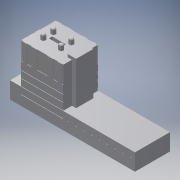
# Autodesk Inventor part: Vertigo
Saved by Autodesk Inventor 2018.3 (Build 223284000, 284)
## iProperties
Created: 2020-12-08
Part Number: Vertigo
Material: Acetal Resin, White
Document SubType Name: Modeling
Designer: daanv
Density: 1.425 g/cm^3
Appearance: Smooth - White
Author: daanv
Autodesk Inventor part; units mm, degrees
note: some values were not read from the file. Chosen so that the rebuilt part matches the saved one: pattern direction of "Rectangular Pattern3".
ref_plane "YZ Plane" through (0, 0, 0) normal (1, 0, 0) x (0, 1, 0)
ref_plane "XZ Plane" through (0, 0, 0) normal (0, 1, 0) x (-1, 0, 0)
ref_plane "XY Plane" through (0, 0, 0) normal (0, 0, 1) x (1, 0, 0)
sketch "Sketch1" plane through (0, 0, 0) normal (0, 0, 1) x (1, 0, 0)
  line L0 (0, 0) -> (100, 0)
  line L1 (100, 0) -> (100, 28.01)
  line L2 (100, 28.01) -> (0, 28.01)
  line L3 (0, 28.01) -> (0, 0)
  dimension "d0" = 100
  dimension "d1" = 28.01
  constraints: 8 end point, 2 parallel, 1 horizontal, 1 perpendicular
  measures "d0" distance of L2.end L1.end
  measures "d1" distance of L1.end L0.end
extrude "Extrusion1" add sketch "Sketch1" along normal blind 13.41
sketch "Sketch2" plane through (0, 0, 13.41) normal (0, 0, 1) x (1, 0, 0)
  line L0 (0, 0) -> (100, 0) projected
  line L1 (100, 0) -> (100, 28.01) projected
  line L2 (100, 28.01) -> (0, 28.01) projected
  line L3 (0, 28.01) -> (0, 0) projected
  line L4 (8.81, 27.7) -> (42.45, 27.7)
  line L5 (42.45, 27.7) -> (42.45, 0.31)
  line L6 (42.45, 0.31) -> (8.81, 0.31)
  line L7 (8.81, 0.31) -> (8.81, 27.7)
  dimension "d4" = 0.31
  dimension "d5" = 0.31
  dimension "d6" = 8.81
  dimension "d7" = 57.55
  dimension "d8" = 33.64
  dimension "d9" = 27.39
  constraints: 8 end point, 2 parallel, 1 horizontal, 1 perpendicular
  measures "d4" distance between parallel lines of L0 L6
  measures "d5" distance between parallel lines of L2 L4
  measures "d6" distance between parallel lines of L7 L3
  measures "d7" distance between parallel lines of L1 L5
  measures "d8" distance of L4.start L4.end
  measures "d9" distance of L4.end L5.end
extrude "Extrusion2" add sketch "Sketch2" along normal blind 31.92 contours L4 L5 L6 L7
sketch "Sketch3" plane through (0, 0, 13.41) normal (0, 0, 1) x (1, 0, 0)
  line L0 (42.45, 27.7) -> (42.45, 0.31) projected
  line L1 (42.45, 0.31) -> (8.81, 0.31) projected
  line L2 (8.81, 27.7) -> (42.45, 27.7) projected
  line L3 (42.45, 20.9) -> (45.8, 20.9)
  line L4 (45.8, 20.9) -> (45.8, 7.11)
  line L5 (45.8, 7.11) -> (42.45, 7.11)
  line L6 (42.45, 7.11) -> (42.45, 20.9)
  dimension "d12" = 6.8
  dimension "d13" = 6.8
  dimension "d14" = 3.35
  constraints: 8 end point, 2 parallel, 1 horizontal, 1 perpendicular, 1 point on line
  measures "d12" distance between parallel lines of L1 L5
  measures "d13" distance between parallel lines of L3 L2
  measures "d14" distance between parallel lines of L4 L0
extrude "Extrusion3" add sketch "Sketch3" along normal blind 34.21
sketch "Sketch4" plane through (42.45, 7.11, 45.33) normal (-1, 0, 0) x (0, 0, 1)
  line L0 (0, 0) -> (0, 13.79) projected
  line L1 (0, 0) -> (2.29, 0) projected
  line L2 (2.29, 13.79) -> (2.29, 0) projected
  line L3 (0, 13.79) -> (2.29, 13.79) projected
  point P0 (-45.33, -7.11)
extrude "Extrusion4" add sketch "Sketch4" along normal blind 3.44
sketch "Sketch5" plane through (0, 0, 0) normal (0, -1, 0) x (1, 0, 0)
  line L0 (100, 0) -> (100, 13.41) projected
  line L1 (0, 13.41) -> (100, 13.41) projected
  line L2 (97.05, 10.28) -> (95.8, 10.28)
  line L3 (95.8, 10.28) -> (95.8, 7.78)
  line L4 (95.8, 7.78) -> (97.05, 7.78)
  line L5 (97.05, 7.78) -> (97.05, 10.28)
  dimension "d19" = 2.5
  dimension "d20" = 1.25
  dimension "d21" = 1.25
  dimension "d22" = 3.13
  dimension "d23" = 2.95
  constraints: 8 end point, 2 parallel, 1 horizontal, 1 perpendicular
  measures "d19" distance of L2.end L3.end
  measures "d20" distance of L3.end L4.end
  measures "d21" distance of L2.start L2.end
  measures "d22" distance between parallel lines of L1 L2
  measures "d23" distance between parallel lines of L0 L5
extrude "Extrusion5" cut sketch "Sketch5" against normal blind 0.31
pattern_linear "Rectangular Pattern1" count 9 spacing 6.25 along (-1, 0, 0) of "Extrusion5"
sketch "Sketch6" plane through (0, 0, 0) normal (0, -1, 0) x (1, 0, 0)
  line L0 (45.8, 7.78) -> (45.8, 10.28) projected
  line L1 (0, 0) -> (100, 0) projected
  line L2 (0, 13.41) -> (100, 13.41) projected
  line L3 (42.45, 10.28) -> (8.49, 10.28)
  line L4 (8.49, 10.28) -> (8.49, 7.78)
  line L5 (8.49, 7.78) -> (42.45, 7.78)
  line L6 (42.45, 7.78) -> (42.45, 10.28)
  dimension "d29" = 3.35
  dimension "d30" = 33.96
  dimension "d31" = 3.13
  dimension "d32" = 7.78
  constraints: 8 end point, 2 parallel, 1 horizontal, 1 perpendicular
  measures "d29" distance between parallel lines of L0 L6
  measures "d30" distance of L4.end L5.end
  measures "d31" distance between parallel lines of L2 L3
  measures "d32" distance between parallel lines of L1 L5
extrude "Extrusion6" cut sketch "Sketch6" against normal blind 0.31
sketch "Sketch7" plane through (0, 28.01, 0) normal (0, 1, 0) x (1, 0, 0)
  line L0 (95.8, -7.78) -> (95.8, -10.28) projected
  line L1 (97.05, -10.28) -> (97.05, -7.78) projected
  line L2 (95.8, -10.28) -> (97.05, -10.28)
  line L3 (97.05, -10.28) -> (97.05, -7.78)
  line L4 (97.05, -7.78) -> (95.8, -7.78)
  line L5 (95.8, -7.78) -> (95.8, -10.28)
  constraints: 8 end point, 2 parallel, 1 horizontal, 1 perpendicular
extrude "Extrusion7" cut sketch "Sketch7" against normal blind 0.31
pattern_linear "Rectangular Pattern2" count 9 spacing 6.25 along (-1, 0, 0) of "Extrusion7"
sketch "Sketch8" plane through (0, 28.01, 0) normal (0, 1, 0) x (1, 0, 0)
  line L0 (8.49, -10.28) -> (42.45, -10.28) projected
  line L1 (42.45, -7.78) -> (8.49, -7.78) projected
  line L2 (42.45, -10.28) -> (8.49, -10.28)
  line L3 (8.49, -10.28) -> (8.49, -7.78)
  line L4 (8.49, -7.78) -> (42.45, -7.78)
  line L5 (42.45, -7.78) -> (42.45, -10.28)
  constraints: 8 end point, 2 parallel, 1 horizontal, 1 perpendicular
extrude "Extrusion8" cut sketch "Sketch8" against normal blind 0.31
sketch "Sketch9" plane through (0, 0, 0) normal (-1, 0, 0) x (0, 0, 1)
  line L0 (0, 28.01) -> (0, 0) projected
  line L1 (0, 28.01) -> (13.41, 28.01) projected
  line L2 (0, 0.7696) -> (5.26, 0.7696)
  line L3 (5.26, 0.7696) -> (5.26, 27.3796)
  line L4 (5.26, 27.3796) -> (2.67, 27.3796)
  line L5 (2.67, 27.3796) -> (2.67, 25.2896)
  line L6 (2.67, 25.2896) -> (0, 0.7696)
  dimension "d42" = 5.26
  dimension "d43" = 26.61
  dimension "d44" = 2.59
  dimension "d45" = 2.09
  constraints: 10 end point, 2 horizontal, 2 perpendicular, 1 point on line
  measures "d42" distance of L2.start L2.end
  measures "d43" distance of L2.end L3.end
  measures "d44" distance of L3.end L4.end
  measures "d45" distance of L4.end L5.end
extrude "Extrusion9" cut sketch "Sketch9" against normal blind 1.25
sketch "Sketch10" plane through (1.25, 0, 0) normal (-1, 0, 0) x (0, 0, 1)
  line L0 (2.67, 27.3796) -> (5.26, 27.3796) projected
  line L1 (2.67, 25.2896) -> (2.67, 27.3796) projected
  line L2 (5.26, 27.3796) -> (2.67, 27.3796)
  line L3 (2.67, 27.3796) -> (2.67, 25.2896)
  line L4 (2.67, 25.2896) -> (5.26, 25.2896)
  line L5 (5.26, 25.2896) -> (5.26, 27.3796)
  point P0 (0, 0)
  constraints: 8 end point, 2 parallel, 1 horizontal, 1 perpendicular
extrude "Extrusion10" cut sketch "Sketch10" against normal blind 1.24
sketch "Sketch11" plane through (8.81, 0.31, 13.41) normal (0, -1, 0) x (1, 0, 0)
  line L0 (33.64, 0) -> (0, 0) projected
  line L1 (0, 0) -> (0, 31.92) projected
  line L2 (33.64, 31.92) -> (33.64, 0) projected
  line L3 (0, 2.5) -> (33.64, 2.5)
  line L4 (33.64, 2.5) -> (33.64, 5.63)
  line L5 (33.64, 5.63) -> (0, 5.63)
  line L6 (0, 5.63) -> (0, 2.5)
  point P0 (-8.81, -13.41)
  dimension "d50" = 3.13
  dimension "d51" = 2.5
  constraints: 8 end point, 2 parallel, 2 point on line, 1 horizontal, 1 perpendicular
  measures "d50" distance of L4.end L3.end
  measures "d51" distance between parallel lines of L0 L3
extrude "Extrusion11" add sketch "Sketch11" along normal blind 0.31 contours L3 L1 L5 L2
pattern_linear "Rectangular Pattern3" count 2 spacing 5.63 along (0, 0, 1) of "Extrusion11"
sketch "Sketch12" plane through (8.81, 0.31, 45.33) normal (0, -1, 0) x (1, 0, 0)
  line L0 (0, -20.66) -> (33.64, -20.66) projected
  line L1 (33.64, -20.66) -> (33.64, 0) projected
  line L2 (0, -20.66) -> (0, 0) projected
  line L3 (0, -18.16) -> (33.64, -18.16)
  line L4 (33.64, -18.16) -> (33.64, -14.09)
  line L5 (33.64, -14.09) -> (0, -14.09)
  line L6 (0, -14.09) -> (0, -18.16)
  point P0 (-8.81, -45.33)
  dimension "d57" = 4.07
  dimension "d58" = 2.5
  constraints: 8 end point, 2 parallel, 2 point on line, 1 horizontal, 1 perpendicular
  measures "d57" distance of L4.end L3.end
  measures "d58" distance between parallel lines of L0 L3
extrude "Extrusion12" add sketch "Sketch12" along normal blind 0.31 contours L2 L5 L1 L3
sketch "Sketch13" plane through (8.81, 0.31, 31.24) normal (0, 0, 1) x (1, 0, 0)
  line L0 (0, 0) -> (33.64, 0) projected
  line L1 (33.64, -0.31) -> (0, -0.31) projected
  line L2 (-8.81, -0.31) -> (91.19, -0.31) projected
  line L3 (1.52, 0) -> (4.62, 0)
  line L4 (4.62, 0) -> (4.62, -0.31)
  line L5 (4.62, -0.31) -> (1.52, -0.31)
  line L6 (1.52, -0.31) -> (1.52, 0)
  line L7 (-0.32, 0) -> (33.64, 0) projected
  line L8 (8.21, 0) -> (12.82, 0)
  line L9 (12.82, 0) -> (12.82, -0.31)
  line L10 (12.82, -0.31) -> (8.21, -0.31)
  line L11 (8.21, -0.31) -> (8.21, 0)
  line L12 (21.12, 0) -> (25.73, 0)
  line L13 (25.73, 0) -> (25.73, -0.31)
  line L14 (25.73, -0.31) -> (21.12, -0.31)
  line L15 (21.12, -0.31) -> (21.12, 0)
  line L16 (29.32, 0) -> (32.42, 0)
  line L17 (32.42, 0) -> (32.42, -0.31)
  line L18 (32.42, -0.31) -> (29.32, -0.31)
  line L19 (29.32, -0.31) -> (29.32, 0)
  dimension "d61" = 3.1
  dimension "d62" = 4.61
  dimension "d63" = 4.61
  dimension "d64" = 3.1
  constraints: 32 end point, 8 parallel, 8 point on line, 4 horizontal, 4 perpendicular
  measures "d61" distance of L4.end L5.end
  measures "d62" distance of L9.end L10.end
  measures "d63" distance of L13.end L14.end
  measures "d64" distance of L17.end L18.end
extrude "Extrusion13" add sketch "Sketch13" along normal blind 14.1 contours L0 L4 L1 L6 | L0 L9 L1 L11 | L0 L13 L1 L15 | L0 L17 L1 L19
sketch "Sketch14" plane through (8.81, 27.7, 13.41) normal (0, 1, 0) x (1, 0, 0)
  line L0 (0, 0) -> (0, -31.92) projected
  line L1 (33.64, -2.5) -> (0, -2.5) projected
  line L2 (33.64, -5.63) -> (0, -5.63) projected
  line L3 (33.64, -2.5) -> (0, -2.5)
  line L4 (0, -2.5) -> (0, -5.63)
  line L5 (0, -5.63) -> (33.64, -5.63)
  line L6 (33.64, -5.63) -> (33.64, -2.5)
  line L7 (0, -8.13) -> (33.64, -8.13) projected
  line L8 (0, -11.26) -> (33.64, -11.26) projected
  line L9 (33.64, -8.13) -> (0, -8.13)
  line L10 (0, -8.13) -> (0, -11.26)
  line L11 (0, -11.26) -> (33.64, -11.26)
  line L12 (33.64, -11.26) -> (33.64, -8.13)
  line L13 (33.64, -13.76) -> (0, -13.76) projected
  line L14 (1.52, -17.83) -> (0, -17.83) projected
  line L15 (33.64, -13.76) -> (0, -13.76)
  line L16 (0, -13.76) -> (0, -17.83)
  line L17 (0, -17.83) -> (33.64, -17.83)
  line L18 (33.64, -17.83) -> (33.64, -13.76)
  point P0 (-8.81, 13.41)
  constraints: 24 end point, 6 parallel, 3 horizontal, 3 perpendicular
extrude "Extrusion14" add sketch "Sketch14" along normal blind 0.31
sketch "Sketch15" plane through (8.81, 27.7, 45.33) normal (0, 1, 0) x (1, 0, 0)
  line L0 (32.42, 14.09) -> (32.42, -0.01) projected
  line L1 (29.32, 14.09) -> (29.32, -0.01) projected
  line L2 (32.42, -0.01) -> (29.32, -0.01)
  line L3 (29.32, -0.01) -> (29.32, 14.09)
  line L4 (29.32, 14.09) -> (32.42, 14.09)
  line L5 (32.42, 14.09) -> (32.42, -0.01)
  line L6 (25.73, 0) -> (25.73, 14.09) projected
  line L7 (21.12, 14.09) -> (21.12, -0.01) projected
  line L8 (25.73, 0) -> (21.12, 0)
  line L9 (21.12, 0) -> (21.12, 14.09)
  line L10 (21.12, 14.09) -> (25.73, 14.09)
  line L11 (25.73, 14.09) -> (25.73, 0)
  line L12 (12.82, 14.09) -> (12.82, -0.01) projected
  line L13 (8.21, 14.09) -> (8.21, -0.01) projected
  line L14 (12.82, -0.01) -> (8.21, -0.01)
  line L15 (8.21, -0.01) -> (8.21, 14.09)
  line L16 (8.21, 14.09) -> (12.82, 14.09)
  line L17 (12.82, 14.09) -> (12.82, -0.01)
  line L18 (1.52, 14.09) -> (1.52, 0) projected
  line L19 (4.62, 14.09) -> (4.62, -0.01) projected
  line L20 (1.52, 0) -> (4.62, 0)
  line L21 (4.62, 0) -> (4.62, 14.09)
  line L22 (4.62, 14.09) -> (1.52, 14.09)
  line L23 (1.52, 14.09) -> (1.52, 0)
  point P0 (-8.81, 45.33)
  constraints: 32 end point, 8 parallel, 4 horizontal, 4 perpendicular
extrude "Extrusion15" add sketch "Sketch15" along normal blind 0.31
sketch "Sketch16" plane through (8.81, 0.31, 13.41) normal (-1, 0, 0) x (0, 0, 1)
  line L0 (17.82, 27.39) -> (0, 27.39)
  line L1 (0, 27.39) -> (0, 0)
  line L2 (0, 0) -> (17.82, 0)
  line L3 (17.82, 0) -> (17.82, 27.39)
  point P0 (-13.41, -0.31)
  constraints: 8 end point, 2 parallel, 1 horizontal, 1 perpendicular
extrude "Extrusion16" add sketch "Sketch16" along normal blind 0.31
sketch "Sketch17" plane through (8.81, 0.31, 45.33) normal (-1, 0, 0) x (0, 0, 1)
  line L0 (0, 27.39) -> (0, 0) projected
  line L1 (-14.09, 27.39) -> (0, 27.39) projected
  line L2 (-14.1, 27.39) -> (-14.1, 0) projected
  line L3 (0, 6.8) -> (0, 20.59) projected
  line L4 (-14.1, 15) -> (0, 15)
  line L5 (0, 15) -> (0, 10.62)
  line L6 (0, 10.62) -> (-14.1, 10.62)
  line L7 (-14.1, 10.62) -> (-14.1, 15)
  line L8 (0, 9.92) -> (-14.1, 9.92)
  line L9 (-14.1, 9.92) -> (-14.1, 5.54)
  line L10 (-14.1, 5.54) -> (0, 5.54)
  line L11 (0, 5.54) -> (0, 9.92)
  line L12 (0, 0) -> (0, 6.8) projected
  line L13 (0, 4.84) -> (-14.1, 4.84)
  line L14 (-14.1, 4.84) -> (-14.1, 0.46)
  line L15 (-14.1, 0.46) -> (0, 0.46)
  line L16 (0, 0.46) -> (0, 4.84)
  point P0 (-45.33, -0.31)
  dimension "d73" = 4.38
  dimension "d74" = 4.38
  dimension "d75" = 4.38
  dimension "d76" = 12.39
  dimension "d77" = 0.7
  dimension "d78" = 0.7
  constraints: 24 end point, 6 parallel, 6 point on line, 3 horizontal, 3 perpendicular
  measures "d73" distance of L4.end L5.end
  measures "d74" distance of L9.end L8.end
  measures "d75" distance of L14.end L13.end
  measures "d76" distance between parallel lines of L1 L4
  measures "d77" distance between parallel lines of L6 L8
  measures "d78" distance between parallel lines of L10 L13
extrude "Extrusion17" add sketch "Sketch17" along normal blind 0.31 contours L0 L6 L2 L4 | L0 L10 L2 L8 | L0 L15 L2 L13
sketch "Sketch18" plane through (0, 0, 45.33) normal (0, 0, 1) x (1, 0, 0)
  line L0 (39.01, 7.11) -> (39.01, 20.9) projected
  line L1 (42.45, 20.9) -> (42.45, 27.7) projected
  line L2 (29.93, 27.7) -> (21.63, 27.7) projected
  line L3 (8.81, 27.7) -> (8.81, 15.31) projected
  line L4 (13.91, 21.01) -> (33.91, 21.01)
  line L5 (33.91, 21.01) -> (33.91, 7.01)
  line L6 (33.91, 7.01) -> (13.91, 7.01)
  line L7 (13.91, 7.01) -> (13.91, 21.01)
  line L8 (16.7794, 19.91) -> (18.5188, 18.6463)
  line L9 (18.5188, 18.6463) -> (17.8544, 16.6015)
  line L10 (17.8544, 16.6015) -> (15.7044, 16.6015)
  line L11 (15.7044, 16.6015) -> (15.04, 18.6463)
  line L12 (15.04, 18.6463) -> (16.7794, 19.91)
  line L13 (32.7788, 18.6463) -> (32.1144, 16.6015)
  line L14 (32.1144, 16.6015) -> (29.9644, 16.6015)
  line L15 (29.9644, 16.6015) -> (29.3, 18.6463)
  line L16 (29.3, 18.6463) -> (31.0394, 19.91)
  line L17 (31.0394, 19.91) -> (32.7788, 18.6463)
  line L18 (16.7794, 11.7685) -> (18.5188, 10.5048)
  line L19 (18.5188, 10.5048) -> (17.8544, 8.46)
  line L20 (17.8544, 8.46) -> (15.7044, 8.46)
  line L21 (15.7044, 8.46) -> (15.04, 10.5048)
  line L22 (15.04, 10.5048) -> (16.7794, 11.7685)
  line L23 (31.0396, 11.7685) -> (32.779, 10.5048)
  line L24 (32.779, 10.5048) -> (32.1146, 8.46)
  line L25 (32.1146, 8.46) -> (29.9646, 8.46)
  line L26 (29.9646, 8.46) -> (29.3002, 10.5048)
  line L27 (29.3002, 10.5048) -> (31.0396, 11.7685)
  line L28 (18.41, 15.31) -> (29.41, 15.31)
  line L29 (29.41, 15.31) -> (29.41, 12.71)
  line L30 (29.41, 12.71) -> (18.41, 12.71)
  line L31 (18.41, 12.71) -> (18.41, 15.31)
  point P0 (8.5, 0.77)
  point P1 (21.63, 0.31)
  point P2 (0, 0)
  point P3 (16.7794, 18.0811)
  point P4 (31.0394, 18.0811)
  point P5 (16.7794, 9.9396)
  point P6 (31.0396, 9.9396)
  dimension "d81" = 33.64
  dimension "d82" = 26.93
  dimension "d83" = 20
  dimension "d84" = 14
  dimension "d85" = 6.69
  dimension "d86" = 6.7
  dimension "d87" = 5.1
  dimension "d88" = 5.1
  dimension "d89" = 2.15
  dimension "d90" = 1.13
  dimension "d91" = 1.1
  dimension "d92" = 2.15
  dimension "d94" = 1.1
  dimension "d95" = 12.11
  dimension "d96" = 1.1312
  dimension "d97" = 2.15
  dimension "d98" = 2.15
  dimension "d99" = 1.45
  dimension "d100" = 1.45
  dimension "d101" = 1.13
  dimension "d102" = 1.131
  dimension "d103" = 4.833
  dimension "d104" = 12.1102
  dimension "d105" = 11
  dimension "d106" = 2.6
  dimension "d107" = 4.5
  dimension "d108" = 5.7
  constraints: 56 end point, 6 horizontal, 4 parallel, 2 perpendicular, 44 other
  measures "d81" distance between parallel lines of L1 L3
  measures "d82" vertical distance of point (8.5, 0.77) L3.start
  measures "d83" distance of L5.end L6.end
  measures "d84" distance of L4.end L5.end
  measures "d85" distance between parallel lines of L2 L4
  measures "d86" distance from line of point (21.63, 0.31) L6
  measures "d87" distance between parallel lines of L3 L7
  measures "d88" distance between parallel lines of L0 L5
  measures "d89" distance of L9.end L10.end
  measures "d90" distance from line of L7 L11.end
  measures "d91" distance from line of L4 L8.start
  measures "d92" distance of L13.end L14.end
  measures "d94" distance from line of L4 L16.end
  measures "d95" distance of L14.end L9.end
  measures "d96" distance from line of L5 L13.start
  measures "d97" distance of L19.end L20.end
  measures "d98" distance of L24.end L25.end
  measures "d99" distance between parallel lines of L6 L25
  measures "d100" distance between parallel lines of L6 L20
  measures "d101" distance from line of L7 L21.end
  measures "d102" distance from line of L5 L23.end
  measures "d103" distance from line of L14 L23.start
  measures "d104" distance of L25.end L19.end
  measures "d105" distance of L28.start L28.end
  measures "d106" distance of L28.end L29.end
  measures "d107" distance between parallel lines of L7 L31
  measures "d108" distance between parallel lines of L6 L30
extrude "Extrusion18" add sketch "Sketch18" along normal blind 4 contours L8 L9 L10 L11 L12 | L13 L14 L15 L16 L17 | L18 L19 L20 L21 L22 | L23 L24 L25 L26 L27
sketch "Sketch19" plane through (0, 0, 45.33) normal (0, 0, 1) x (1, 0, 0)
  line L0 (18.5188, 10.5048) -> (17.8544, 8.46) projected
  line L1 (17.8544, 8.46) -> (15.7044, 8.46) projected
  line L2 (15.7044, 8.46) -> (15.04, 10.5048) projected
  line L3 (15.04, 10.5048) -> (16.7794, 11.7685) projected
  line L4 (16.7794, 11.7685) -> (18.5188, 10.5048) projected
  line L5 (18.5188, 18.6463) -> (17.8544, 16.6015) projected
  line L6 (17.8544, 16.6015) -> (15.7044, 16.6015) projected
  line L7 (15.7044, 16.6015) -> (15.04, 18.6463) projected
  line L8 (15.04, 18.6463) -> (16.7794, 19.91) projected
  line L9 (16.7794, 19.91) -> (18.5188, 18.6463) projected
  line L10 (32.1144, 16.6015) -> (29.9644, 16.6015) projected
  line L11 (29.9644, 16.6015) -> (29.3, 18.6463) projected
  line L12 (29.3, 18.6463) -> (31.0394, 19.91) projected
  line L13 (31.0394, 19.91) -> (32.7788, 18.6463) projected
  line L14 (32.7788, 18.6463) -> (32.1144, 16.6015) projected
  line L15 (32.779, 10.5048) -> (32.1146, 8.46) projected
  line L16 (32.1146, 8.46) -> (29.9646, 8.46) projected
  line L17 (29.9646, 8.46) -> (29.3002, 10.5048) projected
  line L18 (29.3002, 10.5048) -> (31.0396, 11.7685) projected
  line L19 (31.0396, 11.7685) -> (32.779, 10.5048) projected
  line L20 (42.45, 7.11) -> (39.01, 7.11) projected
  line L21 (39.01, 7.11) -> (39.01, 20.9) projected
  line L22 (39.01, 20.9) -> (42.45, 20.9) projected
  line L23 (42.45, 20.9) -> (42.45, 27.7) projected
  line L24 (42.45, 27.7) -> (41.23, 27.7) projected
  line L25 (41.23, 27.7) -> (38.13, 27.7) projected
  line L26 (38.13, 27.7) -> (34.54, 27.7) projected
  line L27 (34.54, 27.7) -> (34.54, 28.01) projected
  line L28 (29.93, 28.01) -> (34.54, 28.01) projected
  line L29 (29.93, 27.7) -> (29.93, 28.01) projected
  line L30 (29.93, 27.7) -> (21.63, 27.7) projected
  line L31 (21.63, 27.7) -> (17.02, 27.7) projected
  line L32 (17.02, 27.7) -> (13.43, 27.7) projected
  line L33 (13.43, 27.7) -> (13.43, 28.01) projected
  line L34 (10.33, 28.01) -> (13.43, 28.01) projected
  line L35 (10.33, 27.7) -> (10.33, 28.01) projected
  line L36 (10.33, 27.7) -> (8.81, 27.7) projected
  line L37 (8.81, 27.7) -> (8.81, 15.31) projected
  line L38 (8.81, 15.31) -> (8.5, 15.31) projected
  line L39 (8.5, 10.93) -> (8.5, 15.31) projected
  line L40 (8.81, 10.93) -> (8.5, 10.93) projected
  line L41 (8.81, 10.93) -> (8.81, 10.23) projected
  line L42 (8.81, 10.23) -> (8.5, 10.23) projected
  line L43 (8.5, 5.85) -> (8.5, 10.23) projected
  line L44 (8.81, 5.85) -> (8.5, 5.85) projected
  line L45 (8.81, 5.85) -> (8.81, 5.15) projected
  line L46 (8.81, 5.15) -> (8.5, 5.15) projected
  line L47 (8.5, 0.77) -> (8.5, 5.15) projected
  line L48 (8.81, 0.77) -> (8.5, 0.77) projected
  line L49 (8.81, 0.77) -> (8.81, 0.31) projected
  line L50 (8.81, 0.31) -> (10.33, 0.31) projected
  line L51 (10.33, 0.31) -> (13.43, 0.31) projected
  line L52 (13.43, 0.31) -> (17.02, 0.31) projected
  line L53 (17.02, 0.31) -> (21.63, 0.31) projected
  line L54 (21.63, 0.31) -> (29.93, 0.31) projected
  line L55 (29.93, 0.31) -> (34.54, 0.31) projected
  line L56 (34.54, 0.31) -> (38.13, 0.31) projected
  line L57 (38.13, 0.31) -> (41.23, 0.31) projected
  line L58 (41.23, 0.31) -> (42.45, 0.31) projected
  line L59 (42.45, 0.31) -> (42.45, 7.11) projected
  line L60 (18.4023, 15.31) -> (29.4023, 15.31)
  line L61 (29.4023, 15.31) -> (29.4023, 12.71)
  line L62 (29.4023, 12.71) -> (18.4023, 12.71)
  line L63 (18.4023, 12.71) -> (18.4023, 15.31)
  point P0 (0, 0)
  dimension "d111" = 11
  dimension "d112" = 2.6
  dimension "d113" = 12.4
  dimension "d114" = 9.5923
  constraints: 8 end point, 2 parallel, 1 horizontal, 1 perpendicular
  measures "d111" distance of L61.end L62.end
  measures "d112" distance of L60.end L61.end
  measures "d113" distance between parallel lines of L54 L62
  measures "d114" distance between parallel lines of L37 L63
extrude "Extrusion19" cut sketch "Sketch18" against normal blind 40 contours L28 L29 L30 L31
chamfer "Chamfer1" distance 0.5 angle 45 20 edges at (15.3722, 9.4824, 49.33) (15.9097, 11.1366, 49.33) (17.6491, 11.1366, 49.33) (18.1866, 9.4824, 49.33) (16.7794, 8.46, 49.33) (16.7794, 16.6015, 49.33) (15.3722, 17.6239, 49.33) (15.9097, 19.2781, 49.33) (18.1866, 17.6239, 49.33) (17.6491, 19.2781, 49.33) (30.1697, 19.2781, 49.33) (31.9091, 19.2781, 49.33) (32.4466, 17.6239, 49.33) (31.0394, 16.6015, 49.33) (29.6322, 17.6239, 49.33) (30.1699, 11.1366, 49.33) (31.9093, 11.1366, 49.33) (32.4468, 9.4824, 49.33) (31.0396, 8.46, 49.33) (29.6324, 9.4824, 49.33)
body "Solid1"
